Autodesk Fusion 360 part; units mm, degrees
(part 2 of 23)
  line L148 (51.3842, 29.2749) -> (51.3842, 29.6644)
  arc A510 (53.5996, 31.1037) -> (53.5996, 31.0529) centre (53.5996, 31.0783) ccw
  line L149 (53.9242, 28.6399) -> (53.9242, 28.2504)
  arc A511 (52.7812, 28.6399) -> (52.7304, 28.6399) centre (52.7558, 28.6399) ccw
  arc A512 (53.9365, 29.8369) -> (53.9119, 29.8813) centre (53.9242, 29.8591) ccw
  arc A513 (53.9496, 28.6399) -> (53.8988, 28.6399) centre (53.9242, 28.6399) ccw
  arc A514 (52.7812, 28.2504) -> (52.7304, 28.2504) centre (52.7558, 28.2504) ccw
  arc A515 (53.9496, 28.2504) -> (53.8988, 28.2504) centre (53.9242, 28.2504) ccw
  arc A516 (37.4142, 29.5233) -> (36.7651, 29.5233) centre (37.0896, 29.5233) ccw
  arc A517 (36.2204, 29.5882) -> (36.2712, 29.5882) centre (36.2458, 29.5882) ccw
  arc A518 (53.8988, 28.2504) -> (53.9496, 28.2504) centre (53.9242, 28.2504) ccw
  arc A519 (36.7651, 29.5882) -> (36.2458, 29.5882) centre (36.5055, 29.5882) ccw
  arc A520 (36.7905, 29.5882) -> (36.7397, 29.5882) centre (36.7651, 29.5882) ccw
  arc A521 (53.9242, 28.6145) -> (53.9242, 28.6653) centre (53.9242, 28.6399) ccw
  line L150 (53.2751, 28.4452) -> (53.2751, 28.6399)
  arc A522 (53.2497, 28.4452) -> (53.3005, 28.4452) centre (53.2751, 28.4452) ccw
  arc A523 (53.6646, 27.9654) -> (53.6646, 28.0162) centre (53.6646, 27.9908) ccw
  arc A524 (37.0967, 28.0882) -> (37.1475, 28.0882) centre (37.1221, 28.0882) ccw
  line L151 (53.9242, 29.21) -> (52.7558, 29.21)
  line L152 (53.9242, 30.4292) -> (52.7558, 30.4292)
  line L153 (52.7558, 29.21) -> (53.9242, 29.8591)
  line L154 (53.9242, 29.8591) -> (52.7558, 29.8591)
  line L155 (53.2751, 28.6399) -> (53.9242, 28.6399)
  arc A525 (52.7558, 29.8845) -> (52.7558, 29.8337) centre (52.7558, 29.8591) ccw
  arc A526 (53.9242, 29.8337) -> (53.9242, 29.8845) centre (53.9242, 29.8591) ccw
  arc A527 (36.2712, 29.5882) -> (36.2204, 29.5882) centre (36.2458, 29.5882) ccw
  arc A528 (53.6646, 28.0162) -> (53.6646, 27.9654) centre (53.6646, 27.9908) ccw
  arc A529 (53.9242, 29.1846) -> (53.9242, 29.2354) centre (53.9242, 29.21) ccw
  line L156 (37.4142, 29.1987) -> (37.4142, 29.5233)
  arc A530 (36.7397, 29.5882) -> (36.7905, 29.5882) centre (36.7651, 29.5882) ccw
  arc A531 (36.7397, 29.5233) -> (36.7905, 29.5233) centre (36.7651, 29.5233) ccw
  line L157 (36.7651, 29.5882) -> (36.7651, 29.3285)
  line L158 (52.7558, 30.4292) -> (52.7558, 30.7537)
  arc A532 (52.7812, 30.7537) -> (52.7304, 30.7537) centre (52.7558, 30.7537) ccw
  arc A533 (36.2204, 29.1987) -> (36.2712, 29.1987) centre (36.2458, 29.1987) ccw
  line L159 (52.7558, 28.2504) -> (52.7558, 28.6399)
  arc A534 (52.7304, 30.4292) -> (52.7812, 30.4292) centre (52.7558, 30.4292) ccw
  line L160 (53.0804, 31.0783) -> (53.5996, 31.0783)
  arc A535 (53.6646, 27.9908) -> (53.9242, 28.2504) centre (53.6646, 28.2504) ccw
  arc A536 (53.2751, 28.6653) -> (53.2751, 28.6145) centre (53.2751, 28.6399) ccw
  arc A537 (52.7558, 30.4546) -> (52.7558, 30.4038) centre (52.7558, 30.4292) ccw
  line L161 (53.6646, 27.9908) -> (53.0154, 27.9908)
  arc A538 (51.3588, 29.2749) -> (51.4096, 29.2749) centre (51.3842, 29.2749) ccw
  line L162 (55.3085, 2.4892) -> (55.9576, 2.4892)
  arc A539 (59.4599, 1.2954) -> (59.4599, 1.3462) centre (59.4599, 1.3208) ccw
  arc A540 (58.1499, 1.5804) -> (58.0991, 1.5804) centre (58.1245, 1.5804) ccw
  line L163 (50.9298, 27.9908) -> (50.9298, 28.7697)
  arc A541 (57.3644, 1.8655) -> (57.3644, 1.8147) centre (57.3644, 1.8401) ccw
  arc A542 (59.4599, 1.3462) -> (59.4599, 1.2954) centre (59.4599, 1.3208) ccw
  arc A543 (58.0991, 1.5804) -> (58.1499, 1.5804) centre (58.1245, 1.5804) ccw
  arc A544 (61.5711, 2.4812) -> (61.5229, 2.4972) centre (61.547, 2.4892) ccw
  arc A545 (55.3085, 2.5146) -> (55.3085, 2.4638) centre (55.3085, 2.4892) ccw
  arc A546 (59.4599, 2.4638) -> (59.4599, 2.5146) centre (59.4599, 2.4892) ccw
  arc A547 (57.3644, 2.4638) -> (57.3644, 2.5146) centre (57.3644, 2.4892) ccw
  arc A548 (55.9576, 2.4638) -> (55.9576, 2.5146) centre (55.9576, 2.4892) ccw
  line L164 (61.1575, 1.3208) -> (61.547, 2.4892)
  arc A549 (59.1354, 2.5146) -> (59.1354, 2.4638) centre (59.1354, 2.4892) ccw
  line L165 (58.6438, 1.3208) -> (58.3842, 1.3208)
  line L166 (57.0399, 1.3208) -> (57.0399, 2.4892)
  arc A550 (58.3842, 1.3462) -> (58.3842, 1.2954) centre (58.3842, 1.3208) ccw
  line L167 (58.3842, 2.4892) -> (58.6438, 2.4892)
  arc A551 (59.1608, 2.4892) -> (59.11, 2.4892) centre (59.1354, 2.4892) ccw
  arc A552 (61.976, 1.3462) -> (61.976, 1.2954) centre (61.976, 1.3208) ccw
  arc A553 (59.4599, 1.9953) -> (59.4599, 1.9445) centre (59.4599, 1.9699) ccw
  line L168 (51.3193, 28.3803) -> (50.5404, 28.3803)
  arc A554 (50.5404, 28.4057) -> (50.5404, 28.3549) centre (50.5404, 28.3803) ccw
  arc A555 (59.4599, 1.9953) -> (59.4599, 1.9445) centre (59.4599, 1.9699) ccw
  arc A556 (61.1334, 1.3288) -> (61.1816, 1.3128) centre (61.1575, 1.3208) ccw
  arc A557 (57.3644, 1.8401) -> (57.3644, 2.4892) centre (57.3644, 2.1646) ccw
  arc A558 (58.6438, 2.4638) -> (58.6438, 2.5146) centre (58.6438, 2.4892) ccw
  arc A559 (62.3005, 1.3208) -> (62.3005, 1.9699) centre (62.3005, 1.6453) ccw
  line L169 (57.0399, 2.4892) -> (57.3644, 2.4892)
  line L170 (59.1354, 2.4892) -> (59.4599, 2.4892)
  arc A560 (62.3005, 1.2954) -> (62.3005, 1.3462) centre (62.3005, 1.3208) ccw
  line L171 (59.1354, 1.3208) -> (59.1354, 2.4892)
  line L172 (59.4599, 1.3208) -> (59.1354, 1.3208)
  arc A561 (59.1354, 1.3462) -> (59.1354, 1.2954) centre (59.1354, 1.3208) ccw
  arc A562 (59.11, 1.3208) -> (59.1608, 1.3208) centre (59.1354, 1.3208) ccw
  line L173 (58.1245, 1.5804) -> (58.1245, 2.2296)
  arc A563 (51.4096, 29.6644) -> (51.3588, 29.6644) centre (51.3842, 29.6644) ccw
  arc A564 (51.3842, 29.6644) -> (51.1246, 29.924) centre (51.1246, 29.6644) ccw
  arc A565 (59.4599, 2.5146) -> (59.4599, 2.4638) centre (59.4599, 2.4892) ccw
  arc A566 (50.9044, 27.9908) -> (50.9552, 27.9908) centre (50.9298, 27.9908) ccw
  arc A567 (58.0991, 2.2296) -> (58.1499, 2.2296) centre (58.1245, 2.2296) ccw
  arc A568 (58.1499, 2.2296) -> (58.0991, 2.2296) centre (58.1245, 2.2296) ccw
  arc A569 (57.0653, 2.4892) -> (57.0145, 2.4892) centre (57.0399, 2.4892) ccw
  arc A570 (60.7921, 2.4972) -> (60.7439, 2.4812) centre (60.768, 2.4892) ccw
  arc A571 (57.0145, 1.3208) -> (57.0653, 1.3208) centre (57.0399, 1.3208) ccw
  arc A572 (50.9552, 28.7697) -> (50.9044, 28.7697) centre (50.9298, 28.7697) ccw
  arc A573 (59.4599, 1.3208) -> (59.4599, 1.9699) centre (59.4599, 1.6453) ccw
  arc A574 (58.3842, 1.2954) -> (58.3842, 1.3462) centre (58.3842, 1.3208) ccw
  arc A575 (59.1354, 1.9953) -> (59.1354, 1.9445) centre (59.1354, 1.9699) ccw
  arc A576 (58.3842, 2.4892) -> (58.1245, 2.2296) centre (58.3842, 2.2295) ccw
  arc A577 (57.3644, 1.8147) -> (57.3644, 1.8655) centre (57.3644, 1.8401) ccw
  arc A578 (55.6076, 1.3208) -> (55.6584, 1.3208) centre (55.633, 1.3208) ccw
  arc A579 (51.3193, 28.3549) -> (51.3193, 28.4057) centre (51.3193, 28.3803) ccw
  arc A580 (58.3842, 2.4638) -> (58.3842, 2.5146) centre (58.3842, 2.4892) ccw
  arc A581 (59.4599, 1.9699) -> (59.4599, 2.4892) centre (59.4599, 2.2296) ccw
  arc A582 (51.3588, 29.6644) -> (51.4096, 29.6644) centre (51.3842, 29.6644) ccw
  arc A583 (59.4599, 1.9445) -> (59.4599, 1.9953) centre (59.4599, 1.9699) ccw
  line L174 (54.4288, 1.5804) -> (54.4288, 2.2296)
  arc A584 (53.4819, 2.5146) -> (53.4819, 2.4638) centre (53.4819, 2.4892) ccw
  line L175 (57.3644, 1.8401) -> (57.0399, 1.8401)
  line L176 (59.1354, 1.9699) -> (59.4599, 1.9699)
  line L177 (60.768, 2.4892) -> (61.1575, 1.3208)
  arc A585 (57.3644, 2.5146) -> (57.3644, 2.4638) centre (57.3644, 2.4892) ccw
  line L178 (6.3585, 1.1938) -> (6.7479, 2.3622)
  arc A586 (57.0399, 1.8655) -> (57.0399, 1.8147) centre (57.0399, 1.8401) ccw
  line L179 (5.969, 2.3622) -> (6.3585, 1.1938)
  arc A587 (13.9023, 1.1938) -> (13.9531, 1.1938) centre (13.9277, 1.1938) ccw
  arc A588 (12.9892, 1.1858) -> (13.0374, 1.2018) centre (13.0133, 1.1938) ccw
  arc A589 (14.0575, 1.1684) -> (14.0575, 1.2192) centre (14.0575, 1.1938) ccw
  line L180 (5.54, 1.4534) -> (5.54, 1.5833)
  line L181 (13.7978, 1.1938) -> (14.0575, 1.1938)
  arc A590 (62.3654, 1.9445) -> (62.3654, 1.9953) centre (62.3654, 1.9699) ccw
  arc A591 (4.8655, 1.8429) -> (4.9163, 1.8429) centre (4.8909, 1.8429) ccw
  arc A592 (13.4268, 2.3542) -> (13.3786, 2.3702) centre (13.4027, 2.3622) ccw
  line L182 (13.7978, 2.3622) -> (14.0575, 2.3622)
  arc A593 (57.0399, 2.5146) -> (57.0399, 2.4638) centre (57.0399, 2.4892) ccw
  arc A594 (14.0575, 2.3368) -> (14.0575, 2.3876) centre (14.0575, 2.3622) ccw
  line L183 (4.8909, 1.8429) -> (4.8909, 2.3622)
  arc A595 (5.2804, 1.8683) -> (5.2804, 1.8175) centre (5.2804, 1.8429) ccw
  arc A596 (5.5654, 1.4534) -> (5.5146, 1.4534) centre (5.54, 1.4534) ccw
  arc A597 (5.54, 2.3368) -> (5.54, 2.3876) centre (5.54, 2.3622) ccw
  line L184 (14.5556, 1.1938) -> (14.5556, 2.3622)
  arc A598 (4.8909, 1.2192) -> (4.8909, 1.1684) centre (4.8909, 1.1938) ccw
  arc A599 (14.581, 2.3622) -> (14.5302, 2.3622) centre (14.5556, 2.3622) ccw
  line L185 (61.976, 1.3208) -> (62.3005, 1.3208)
  arc A600 (5.5146, 1.5833) -> (5.5654, 1.5833) centre (5.54, 1.5833) ccw
  line L186 (4.8909, 2.3622) -> (5.54, 2.3622)
  arc A601 (5.2804, 1.8175) -> (5.2804, 1.8683) centre (5.2804, 1.8429) ccw
  arc A602 (62.1058, 1.9953) -> (62.1058, 1.9445) centre (62.1058, 1.9699) ccw
  line L187 (13.9277, 2.3622) -> (13.9277, 1.1938)
  arc A603 (62.3654, 1.9953) -> (62.3654, 1.9445) centre (62.3654, 1.9699) ccw
  arc A604 (61.976, 2.5146) -> (61.976, 2.4638) centre (61.976, 2.4892) ccw
  arc A605 (5.2804, 1.2192) -> (5.2804, 1.1684) centre (5.2804, 1.1938) ccw
  arc A606 (5.2804, 1.1938) -> (5.54, 1.4534) centre (5.2804, 1.4534) ccw
  line L188 (3.9963, 1.2587) -> (3.9963, 2.0376)
  arc A607 (3.6068, 1.6736) -> (3.6068, 1.6228) centre (3.6068, 1.6482) ccw
  arc A608 (58.6438, 1.2954) -> (58.6438, 1.3462) centre (58.6438, 1.3208) ccw
  arc A609 (4.8909, 1.8683) -> (4.8909, 1.8175) centre (4.8909, 1.8429) ccw
  arc A610 (6.3344, 1.1858) -> (6.3826, 1.2018) centre (6.3585, 1.1938) ccw
  arc A611 (13.7978, 1.2192) -> (13.7978, 1.1684) centre (13.7978, 1.1938) ccw
  arc A612 (5.54, 1.5833) -> (5.2804, 1.8429) centre (5.2804, 1.5833) ccw
  arc A613 (12.6479, 2.3702) -> (12.5997, 2.3542) centre (12.6238, 2.3622) ccw
  arc A614 (14.5778, 2.3745) -> (14.5334, 2.3499) centre (14.5556, 2.3622) ccw
  arc A615 (5.5146, 1.4534) -> (5.5654, 1.4534) centre (5.54, 1.4534) ccw
  line L189 (61.976, 2.4892) -> (62.3654, 2.4892)
  arc A616 (6.772, 2.3542) -> (6.7238, 2.3702) centre (6.7479, 2.3622) ccw
  arc A617 (5.2804, 1.1684) -> (5.2804, 1.2192) centre (5.2804, 1.1938) ccw
  line L190 (13.0133, 1.1938) -> (13.4027, 2.3622)
  arc A618 (61.1334, 1.3128) -> (61.1816, 1.3288) centre (61.1575, 1.3208) ccw
  arc A619 (4.0217, 2.0376) -> (3.9709, 2.0376) centre (3.9963, 2.0376) ccw
  arc A620 (4.9163, 2.3622) -> (4.8655, 2.3622) centre (4.8909, 2.3622) ccw
  arc A621 (4.3857, 1.6228) -> (4.3857, 1.6736) centre (4.3857, 1.6482) ccw
  arc A622 (5.5654, 1.5833) -> (5.5146, 1.5833) centre (5.54, 1.5833) ccw
  arc A623 (58.1245, 1.5804) -> (58.3842, 1.3208) centre (58.3842, 1.5805) ccw
  arc A624 (62.3005, 1.9953) -> (62.3005, 1.9445) centre (62.3005, 1.9699) ccw
  arc A625 (4.8909, 2.3876) -> (4.8909, 2.3368) centre (4.8909, 2.3622) ccw
  arc A626 (62.3654, 2.4638) -> (62.3654, 2.5146) centre (62.3654, 2.4892) ccw
  arc A627 (58.3842, 2.5146) -> (58.3842, 2.4638) centre (58.3842, 2.4892) ccw
  arc A628 (3.9709, 1.2587) -> (4.0217, 1.2587) centre (3.9963, 1.2587) ccw
  arc A629 (5.9931, 2.3702) -> (5.9449, 2.3542) centre (5.969, 2.3622) ccw
  line L191 (3.6068, 1.6482) -> (4.3857, 1.6482)
  arc A630 (6.3344, 1.2018) -> (6.3826, 1.1858) centre (6.3585, 1.1938) ccw
  arc A631 (62.3005, 1.3462) -> (62.3005, 1.2954) centre (62.3005, 1.3208) ccw
  arc A632 (62.3654, 1.9699) -> (62.3654, 2.4892) centre (62.3654, 2.2296) ccw
  line L192 (4.8909, 1.1938) -> (5.2804, 1.1938)
  arc A633 (12.9892, 1.2018) -> (13.0374, 1.1858) centre (13.0133, 1.1938) ccw
  line L193 (5.2804, 1.8429) -> (4.8909, 1.8429)
  arc A634 (40.3154, 19.1262) -> (40.3154, 19.0754) centre (40.3154, 19.1008) ccw
  arc A635 (41.2496, 19.7499) -> (41.1988, 19.7499) centre (41.2242, 19.7499) ccw
  arc A636 (22.7951, 20.3595) -> (22.7951, 20.4103) centre (22.7951, 20.3849) ccw
  arc A637 (15.1793, 1.1938) -> (15.2301, 1.1938) centre (15.2047, 1.1938) ccw
  arc A638 (13.7978, 2.3876) -> (13.7978, 2.3368) centre (13.7978, 2.3622) ccw
  line L194 (40.0558, 20.32) -> (41.2242, 20.9691)
  arc A639 (40.5497, 19.5552) -> (40.6005, 19.5552) centre (40.5751, 19.5552) ccw
  arc A640 (23.4696, 20.7744) -> (23.4188, 20.7744) centre (23.4442, 20.7744) ccw
  arc A641 (40.3154, 19.0754) -> (40.3154, 19.1262) centre (40.3154, 19.1008) ccw
  arc A642 (40.9646, 19.1008) -> (41.2242, 19.3604) centre (40.9646, 19.3604) ccw
  arc A643 (23.4362, 21.8284) -> (23.4522, 21.8766) centre (23.4442, 21.8525) ccw
  line L195 (41.2242, 20.9691) -> (40.0558, 20.9691)
  arc A644 (22.6004, 19.5157) -> (22.6004, 19.4649) centre (22.6004, 19.4903) ccw
  line L196 (22.7951, 20.3849) -> (22.2758, 20.3849)
  line L197 (22.9898, 19.1008) -> (22.9898, 19.8797)
  line L198 (14.5556, 2.3622) -> (15.2047, 1.1938)
  arc A645 (40.0558, 20.9945) -> (40.0558, 20.9437) centre (40.0558, 20.9691) ccw
  arc A646 (41.2242, 19.7245) -> (41.2242, 19.7753) centre (41.2242, 19.7499) ccw
  arc A647 (23.4188, 20.7744) -> (23.4696, 20.7744) centre (23.4442, 20.7744) ccw
  arc A648 (40.0558, 19.3604) -> (40.3154, 19.1008) centre (40.3154, 19.3604) ccw
  line L199 (23.1846, 21.034) -> (23.0547, 21.034)
  arc A649 (40.0812, 19.7499) -> (40.0304, 19.7499) centre (40.0558, 19.7499) ccw
  arc A650 (40.0304, 19.3604) -> (40.0812, 19.3604) centre (40.0558, 19.3604) ccw
  arc A651 (23.4188, 20.3849) -> (23.4696, 20.3849) centre (23.4442, 20.3849) ccw
  arc A652 (41.2496, 19.3604) -> (41.1988, 19.3604) centre (41.2242, 19.3604) ccw
  arc A653 (40.9646, 19.1262) -> (40.9646, 19.0754) centre (40.9646, 19.1008) ccw
  arc A654 (40.0812, 19.3604) -> (40.0304, 19.3604) centre (40.0558, 19.3604) ccw
  arc A655 (23.1846, 21.0086) -> (23.1846, 21.0594) centre (23.1846, 21.034) ccw
  arc A656 (22.2838, 22.266) -> (22.2678, 22.2178) centre (22.2758, 22.2419) ccw
  arc A657 (22.3012, 21.034) -> (22.2504, 21.034) centre (22.2758, 21.034) ccw
  arc A658 (40.9646, 19.0754) -> (40.9646, 19.1262) centre (40.9646, 19.1008) ccw
  line L200 (41.2242, 20.32) -> (40.0558, 20.32)
  arc A659 (22.8205, 20.7744) -> (22.7697, 20.7744) centre (22.7951, 20.7744) ccw
  arc A660 (22.2504, 20.3849) -> (22.3012, 20.3849) centre (22.2758, 20.3849) ccw
  arc A661 (22.2758, 20.4103) -> (22.2758, 20.3595) centre (22.2758, 20.3849) ccw
  arc A662 (23.1846, 21.0594) -> (23.1846, 21.0086) centre (23.1846, 21.034) ccw
  arc A663 (22.7697, 20.3849) -> (22.8205, 20.3849) centre (22.7951, 20.3849) ccw
  arc A664 (14.5302, 1.1938) -> (14.581, 1.1938) centre (14.5556, 1.1938) ccw
  arc A665 (62.3654, 2.5146) -> (62.3654, 2.4638) centre (62.3654, 2.4892) ccw
  line L201 (40.5751, 19.5552) -> (40.5751, 19.7499)
  arc A666 (15.2301, 2.3622) -> (15.1793, 2.3622) centre (15.2047, 2.3622) ccw
  arc A667 (22.9644, 19.1008) -> (23.0152, 19.1008) centre (22.9898, 19.1008) ccw
  arc A668 (23.4522, 21.8284) -> (23.4362, 21.8766) centre (23.4442, 21.8525) ccw
  arc A669 (40.5751, 19.7753) -> (40.5751, 19.7245) centre (40.5751, 19.7499) ccw
  line L202 (40.0558, 19.3604) -> (40.0558, 19.7499)
  line L203 (40.9646, 19.1008) -> (40.3154, 19.1008)
  line L204 (23.4442, 21.8525) -> (22.2758, 22.2419)
  arc A670 (22.7697, 20.7744) -> (22.8205, 20.7744) centre (22.7951, 20.7744) ccw
  arc A671 (40.6005, 19.7499) -> (40.5497, 19.7499) centre (40.5751, 19.7499) ccw
  line L205 (62.3654, 1.9699) -> (62.1058, 1.9699)
  arc A672 (23.0547, 21.0594) -> (23.0547, 21.0086) centre (23.0547, 21.034) ccw
  arc A673 (41.1988, 19.3604) -> (41.2496, 19.3604) centre (41.2242, 19.3604) ccw
  arc A674 (40.0435, 20.3422) -> (40.0681, 20.2978) centre (40.0558, 20.32) ccw
  line L206 (22.2758, 20.3849) -> (22.2758, 21.034)
  arc A675 (13.9531, 2.3622) -> (13.9023, 2.3622) centre (13.9277, 2.3622) ccw
  line L207 (23.3793, 19.4903) -> (22.6004, 19.4903)
  line L208 (23.4442, 20.3849) -> (23.4442, 20.7744)
  line L209 (12.6238, 2.3622) -> (13.0133, 1.1938)
  line L210 (15.2047, 1.1938) -> (15.2047, 2.3622)
  line L211 (41.2242, 19.7499) -> (41.2242, 19.3604)
  arc A676 (22.2678, 21.4871) -> (22.2838, 21.4389) centre (22.2758, 21.463) ccw
  arc A677 (15.1825, 1.1815) -> (15.2269, 1.2061) centre (15.2047, 1.1938) ccw
  arc A678 (23.4442, 20.7744) -> (23.1846, 21.034) centre (23.1846, 20.7744) ccw
  line L212 (22.2758, 21.463) -> (23.4442, 21.8525)
  arc A679 (41.1988, 52.5018) -> (41.2496, 52.5018) centre (41.2242, 52.5018) ccw
  line L213 (27.1893, 28.3803) -> (26.4104, 28.3803)
  line L214 (28.9504, 31.0783) -> (29.4696, 31.0783)
  arc A680 (24.8035, 54.4558) -> (24.8281, 54.4114) centre (24.8158, 54.4336) ccw
  arc A681 (24.8158, 55.1081) -> (24.8158, 55.0573) centre (24.8158, 55.0827) ccw
  arc A682 (27.2796, 29.6644) -> (27.2288, 29.6644) centre (27.2542, 29.6644) ccw
  line L215 (27.2542, 29.2749) -> (27.2542, 29.6644)
  arc A683 (27.2288, 29.2749) -> (27.2796, 29.2749) centre (27.2542, 29.2749) ccw
  arc A684 (27.2542, 29.6644) -> (26.9946, 29.924) centre (26.9946, 29.6644) ccw
  arc A685 (25.9842, 55.0573) -> (25.9842, 55.1081) centre (25.9842, 55.0827) ccw
  arc A686 (26.8252, 28.7697) -> (26.7744, 28.7697) centre (26.7998, 28.7697) ccw
  arc A687 (26.4104, 28.4057) -> (26.4104, 28.3549) centre (26.4104, 28.3803) ccw
  line L216 (26.9946, 29.924) -> (26.8647, 29.924)
  arc A688 (26.9946, 29.9494) -> (26.9946, 29.8986) centre (26.9946, 29.924) ccw
  line L217 (25.9842, 55.0827) -> (24.8158, 55.0827)
  line L218 (29.5346, 27.9908) -> (28.8854, 27.9908)
  arc A689 (26.0858, 29.3003) -> (26.0858, 29.2495) centre (26.0858, 29.2749) ccw
  arc A690 (40.2956, 53.667) -> (40.3353, 53.6988) centre (40.3154, 53.6829) ccw
  arc A691 (26.0938, 31.156) -> (26.0778, 31.1078) centre (26.0858, 31.1319) ccw
  arc A692 (29.5346, 28.0162) -> (29.5346, 27.9654) centre (29.5346, 27.9908) ccw
  line L219 (26.7998, 27.9908) -> (26.7998, 28.7697)
  arc A693 (27.1893, 28.3549) -> (27.1893, 28.4057) centre (27.1893, 28.3803) ccw
  arc A694 (26.7744, 27.9908) -> (26.8252, 27.9908) centre (26.7998, 27.9908) ccw
  arc A695 (27.2462, 30.7184) -> (27.2622, 30.7666) centre (27.2542, 30.7425) ccw
  arc A696 (27.2288, 29.6644) -> (27.2796, 29.6644) centre (27.2542, 29.6644) ccw
  arc A697 (25.9965, 55.0605) -> (25.9719, 55.1049) centre (25.9842, 55.0827) ccw
  arc A698 (40.0756, 54.0233) -> (40.036, 53.9916) centre (40.0558, 54.0075) ccw
  line L220 (33.6042, 53.6829) -> (33.6042, 54.332)
  arc A699 (41.2496, 52.8264) -> (41.1988, 52.8264) centre (41.2242, 52.8264) ccw
  arc A700 (29.1197, 28.4452) -> (29.1705, 28.4452) centre (29.1451, 28.4452) ccw
  line L221 (32.4358, 52.5018) -> (32.4358, 52.8264)
  line L222 (33.6042, 52.8264) -> (33.6042, 52.5018)
  arc A701 (33.6042, 55.1504) -> (32.9551, 55.1504) centre (33.2797, 55.1504) ccw
  arc A702 (32.9297, 55.1504) -> (32.9805, 55.1504) centre (32.9551, 55.1504) ccw
  arc A703 (40.2098, 54.8992) -> (40.2263, 54.9473) centre (40.2181, 54.9233) ccw
  line L223 (32.4358, 54.8259) -> (32.4358, 55.2154)
  line L224 (36.1442, 52.5018) -> (34.9758, 52.5018)
  arc A704 (32.4104, 55.2154) -> (32.4612, 55.2154) centre (32.4358, 55.2154) ccw
  arc A705 (36.1442, 52.4764) -> (36.1442, 52.5272) centre (36.1442, 52.5018) ccw
  arc A706 (40.0558, 54.0329) -> (40.0558, 53.9821) centre (40.0558, 54.0075) ccw
  arc A707 (33.2796, 53.1255) -> (33.2796, 53.1763) centre (33.2796, 53.1509) ccw
  arc A708 (32.7604, 53.1763) -> (32.7604, 53.1255) centre (32.7604, 53.1509) ccw
  arc A709 (33.2796, 53.1763) -> (33.2796, 53.1255) centre (33.2796, 53.1509) ccw
  arc A710 (33.5788, 52.8264) -> (33.6296, 52.8264) centre (33.6042, 52.8264) ccw
  arc A711 (32.4556, 54.0233) -> (32.416, 53.9916) centre (32.4358, 54.0075) ccw
  arc A712 (33.6296, 55.1504) -> (33.5788, 55.1504) centre (33.6042, 55.1504) ccw
  arc A713 (26.8647, 29.924) -> (26.6051, 29.6644) centre (26.8647, 29.6644) ccw
  arc A714 (32.4104, 52.5018) -> (32.4612, 52.5018) centre (32.4358, 52.5018) ccw
  arc A715 (40.0812, 55.1504) -> (40.0304, 55.1504) centre (40.0558, 55.1504) ccw
  arc A716 (32.4612, 52.8264) -> (32.4104, 52.8264) centre (32.4358, 52.8264) ccw
  line L225 (32.7604, 53.1509) -> (33.2796, 53.1509)
  line L226 (32.4358, 54.0075) -> (33.6042, 54.0075)
  line L227 (41.2242, 53.6829) -> (41.2242, 54.332)
  arc A717 (33.6296, 54.332) -> (33.5788, 54.332) centre (33.6042, 54.332) ccw
  arc A718 (32.4104, 54.8259) -> (32.4612, 54.8259) centre (32.4358, 54.8259) ccw
  arc A719 (40.2181, 55.3776) -> (40.0558, 55.1504) centre (40.296, 55.1504) ccw
  arc A720 (33.5788, 52.5018) -> (33.6296, 52.5018) centre (33.6042, 52.5018) ccw
  arc A721 (32.9551, 55.2154) -> (32.4358, 55.2154) centre (32.6955, 55.2154) ccw
  line L228 (33.6042, 54.8259) -> (33.6042, 55.1504)
  line L229 (40.3154, 53.6829) -> (40.0558, 54.0075)
  line L230 (40.0558, 54.0075) -> (41.2242, 54.0075)
  arc A722 (33.6042, 52.4764) -> (33.6042, 52.5272) centre (33.6042, 52.5018) ccw
  arc A723 (33.5788, 54.8259) -> (33.6296, 54.8259) centre (33.6042, 54.8259) ccw
  arc A724 (32.4358, 52.5272) -> (32.4358, 52.4764) centre (32.4358, 52.5018) ccw
  arc A725 (32.9297, 55.2154) -> (32.9805, 55.2154) centre (32.9551, 55.2154) ccw
  arc A726 (41.2242, 53.9821) -> (41.2242, 54.0329) centre (41.2242, 54.0075) ccw
  arc A727 (33.5788, 55.1504) -> (33.6296, 55.1504) centre (33.6042, 55.1504) ccw
  arc A728 (54.4034, 1.5804) -> (54.4542, 1.5804) centre (54.4288, 1.5804) ccw
  arc A729 (32.9297, 54.9557) -> (32.9805, 54.9557) centre (32.9551, 54.9557) ccw
  arc A730 (32.4104, 52.8264) -> (32.4612, 52.8264) centre (32.4358, 52.8264) ccw
  arc A731 (34.9758, 52.5272) -> (34.9758, 52.4764) centre (34.9758, 52.5018) ccw
  arc A732 (32.4612, 55.2154) -> (32.4104, 55.2154) centre (32.4358, 55.2154) ccw
  arc A733 (40.64, 54.8005) -> (40.64, 54.8513) centre (40.64, 54.8259) ccw
  arc A734 (29.7942, 28.6145) -> (29.7942, 28.6653) centre (29.7942, 28.6399) ccw
  arc A735 (32.7604, 53.1255) -> (32.7604, 53.1763) centre (32.7604, 53.1509) ccw
  arc A736 (32.6756, 53.667) -> (32.7153, 53.6988) centre (32.6955, 53.6829) ccw
  arc A737 (32.4358, 54.0329) -> (32.4358, 53.9821) centre (32.4358, 54.0075) ccw
  arc A738 (41.2496, 54.332) -> (41.1988, 54.332) centre (41.2242, 54.332) ccw
  arc A739 (40.0558, 55.1504) -> (40.2181, 54.9233) centre (40.2959, 55.1504) ccw
  arc A740 (33.6296, 52.8264) -> (33.5788, 52.8264) centre (33.6042, 52.8264) ccw
  line L231 (32.6954, 53.6829) -> (32.4358, 54.0075)
  arc A741 (40.2181, 54.9233) -> (40.64, 54.8259) centre (40.6401, 55.7886) ccw
  arc A742 (41.1988, 53.6829) -> (41.2496, 53.6829) centre (41.2242, 53.6829) ccw
  arc A743 (26.1112, 29.924) -> (26.0604, 29.924) centre (26.0858, 29.924) ccw
  arc A744 (32.7604, 53.1509) -> (32.4358, 52.8264) centre (32.7604, 52.8263) ccw
  arc A745 (33.6042, 52.8264) -> (33.2796, 53.1509) centre (33.2796, 52.8263) ccw
  arc A746 (40.2292, 54.9461) -> (40.2069, 54.9004) centre (40.2181, 54.9233) ccw
  arc A747 (33.6042, 53.9821) -> (33.6042, 54.0329) centre (33.6042, 54.0075) ccw
  arc A748 (32.9805, 55.2154) -> (32.9297, 55.2154) centre (32.9551, 55.2154) ccw
  arc A749 (33.5788, 53.6829) -> (33.6296, 53.6829) centre (33.6042, 53.6829) ccw
  line L232 (32.9551, 55.2154) -> (32.9551, 54.9557)
  line L233 (36.1442, 52.8264) -> (36.1442, 52.5018)
  line L234 (34.9758, 52.5018) -> (34.9758, 52.8264)
  arc A750 (36.1696, 52.8264) -> (36.1188, 52.8264) centre (36.1442, 52.8264) ccw
  arc A751 (36.1277, 54.8065) -> (36.1607, 54.8452) centre (36.1442, 54.8258) ccw
  arc A752 (37.8404, 53.1509) -> (37.5158, 52.8264) centre (37.8404, 52.8263) ccw
  arc A753 (36.1442, 52.8264) -> (35.8196, 53.1509) centre (35.8196, 52.8263) ccw
  arc A754 (34.9956, 54.0233) -> (34.956, 53.9916) centre (34.9758, 54.0074) ccw
  arc A755 (38.3596, 53.1763) -> (38.3596, 53.1255) centre (38.3596, 53.1509) ccw
  arc A756 (35.3004, 53.1509) -> (34.9758, 52.8264) centre (35.3004, 52.8263) ccw
  arc A757 (38.3596, 53.1255) -> (38.3596, 53.1763) centre (38.3596, 53.1509) ccw
  arc A758 (38.6842, 53.9821) -> (38.6842, 54.0329) centre (38.6842, 54.0075) ccw
  arc A759 (34.9504, 52.8264) -> (35.0012, 52.8264) centre (34.9758, 52.8264) ccw
  line L235 (35.4951, 55.3776) -> (36.1442, 54.8259)
  line L236 (37.7754, 54.8259) -> (37.5158, 55.1504)
  line L237 (35.3004, 53.1509) -> (35.8196, 53.1509)
  line L238 (37.5158, 52.5018) -> (37.5158, 52.8264)
  arc A760 (35.2679, 55.5004) -> (35.2679, 55.4496) centre (35.2679, 55.475) ccw
  arc A761 (36.1442, 53.9821) -> (36.1442, 54.0329) centre (36.1442, 54.0075) ccw
  arc A762 (37.5412, 52.8264) -> (37.4904, 52.8264) centre (37.5158, 52.8264) ccw
  line L239 (36.1442, 53.6829) -> (36.1442, 54.332)
  arc A763 (35.3004, 53.1763) -> (35.3004, 53.1255) centre (35.3004, 53.1509) ccw
  arc A764 (36.1188, 52.5018) -> (36.1696, 52.5018) centre (36.1442, 52.5018) ccw
  arc A765 (37.4904, 52.8264) -> (37.5412, 52.8264) centre (37.5158, 52.8264) ccw
  line L240 (38.6842, 52.8264) -> (38.6842, 52.5018)
  arc A766 (35.5115, 55.397) -> (35.4786, 55.3583) centre (35.495, 55.3777) ccw
  arc A767 (37.4904, 52.5018) -> (37.5412, 52.5018) centre (37.5158, 52.5018) ccw
  arc A768 (38.6588, 52.5018) -> (38.7096, 52.5018) centre (38.6842, 52.5018) ccw
  line L241 (37.5158, 54.0075) -> (38.6842, 54.0075)
  arc A769 (37.8404, 53.1255) -> (37.8404, 53.1763) centre (37.8404, 53.1509) ccw
  arc A770 (35.4951, 55.3776) -> (35.2679, 55.475) centre (35.2679, 55.1613) ccw
  line L242 (35.2354, 53.6829) -> (34.9758, 54.0075)
  arc A771 (38.6842, 52.4764) -> (38.6842, 52.5272) centre (38.6842, 52.5018) ccw
  arc A772 (37.8404, 53.1763) -> (37.8404, 53.1255) centre (37.8404, 53.1509) ccw
  arc A773 (35.8196, 53.1255) -> (35.8196, 53.1763) centre (35.8196, 53.1509) ccw
  arc A774 (36.1696, 54.332) -> (36.1188, 54.332) centre (36.1442, 54.332) ccw
  arc A775 (34.9504, 55.1829) -> (35.0012, 55.1829) centre (34.9758, 55.1829) ccw
  arc A776 (34.9758, 55.1829) -> (35.2354, 54.8259) centre (35.351, 55.1829) ccw
  arc A777 (34.9504, 52.5018) -> (35.0012, 52.5018) centre (34.9758, 52.5018) ccw
  line L243 (36.1442, 54.8259) -> (36.1442, 55.475)
  arc A778 (35.8196, 53.1763) -> (35.8196, 53.1255) centre (35.8196, 53.1509) ccw
  arc A779 (36.1188, 54.8259) -> (36.1696, 54.8259) centre (36.1442, 54.8259) ccw
  arc A780 (34.9758, 54.0329) -> (34.9758, 53.9821) centre (34.9758, 54.0075) ccw
  line L244 (34.9758, 54.0075) -> (36.1442, 54.0075)
  arc A781 (35.2679, 55.4496) -> (35.2679, 55.5004) centre (35.2679, 55.475) ccw
  arc A782 (36.1696, 55.475) -> (36.1188, 55.475) centre (36.1442, 55.475) ccw
  line L245 (38.6842, 52.5018) -> (37.5158, 52.5018)
  arc A783 (35.0012, 55.1829) -> (34.9504, 55.1829) centre (34.9758, 55.1829) ccw
  arc A784 (36.1188, 52.8264) -> (36.1696, 52.8264) centre (36.1442, 52.8264) ccw
  arc A785 (35.0012, 52.8264) -> (34.9504, 52.8264) centre (34.9758, 52.8264) ccw
  arc A786 (35.3004, 53.1255) -> (35.3004, 53.1763) centre (35.3004, 53.1509) ccw
  arc A787 (35.2679, 55.475) -> (34.9758, 55.1829) centre (35.2679, 55.1829) ccw
  arc A788 (35.4767, 55.3601) -> (35.5135, 55.3952) centre (35.4951, 55.3777) ccw
  arc A789 (37.5158, 52.5272) -> (37.5158, 52.4764) centre (37.5158, 52.5018) ccw
  arc A790 (36.1188, 53.6829) -> (36.1696, 53.6829) centre (36.1442, 53.6829) ccw
  line L246 (37.8404, 53.1509) -> (38.3596, 53.1509)
  arc A791 (38.7096, 52.8264) -> (38.6588, 52.8264) centre (38.6842, 52.8264) ccw
  arc A792 (38.6588, 52.8264) -> (38.7096, 52.8264) centre (38.6842, 52.8264) ccw
  arc A793 (38.6842, 52.8264) -> (38.3596, 53.1509) centre (38.3596, 52.8263) ccw
  arc A794 (37.5356, 54.0233) -> (37.496, 53.9916) centre (37.5158, 54.0074) ccw
  line L247 (37.7754, 53.6829) -> (37.5158, 54.0075)
  arc A795 (37.7556, 53.667) -> (37.7953, 53.6988) centre (37.7754, 53.6829) ccw
  arc A796 (35.2156, 53.667) -> (35.2553, 53.6988) centre (35.2355, 53.6829) ccw
  arc A797 (38.6588, 53.6829) -> (38.7096, 53.6829) centre (38.6842, 53.6829) ccw
  arc A798 (35.2276, 54.8017) -> (35.2433, 54.8501) centre (35.2355, 54.8259) ccw
  line L248 (37.5158, 55.1504) -> (38.6842, 55.1504)
  arc A799 (37.5158, 55.1758) -> (37.5158, 55.125) centre (37.5158, 55.1504) ccw
  arc A800 (38.7096, 54.332) -> (38.6588, 54.332) centre (38.6842, 54.332) ccw
  arc A801 (37.5356, 55.1663) -> (37.496, 55.1346) centre (37.5158, 55.1504) ccw
  arc A802 (37.7556, 54.81) -> (37.7953, 54.8418) centre (37.7754, 54.8259) ccw
  arc A803 (38.6842, 55.125) -> (38.6842, 55.1758) centre (38.6842, 55.1504) ccw
  line L249 (38.6842, 53.6829) -> (38.6842, 54.332)
  arc A804 (37.5158, 54.0329) -> (37.5158, 53.9821) centre (37.5158, 54.0075) ccw
  line L250 (41.2242, 52.5018) -> (40.0558, 52.5018)
  arc A805 (33.6804, 29.5557) -> (33.7312, 29.5557) centre (33.7058, 29.5557) ccw
  arc A806 (40.3804, 53.1255) -> (40.3804, 53.1763) centre (40.3804, 53.1509) ccw
  arc A807 (33.9979, 29.8478) -> (33.7058, 29.5557) centre (33.9979, 29.5557) ccw
  arc A808 (34.5567, 28.0882) -> (34.6075, 28.0882) centre (34.5821, 28.0882) ccw
  line L251 (38.6842, 54.8259) -> (38.6842, 55.475)
  line L252 (37.4974, 2.4892) -> (37.4974, 1.3208)
  arc A809 (38.6588, 54.8259) -> (38.7096, 54.8259) centre (38.6842, 54.8259) ccw
  arc A810 (40.0812, 52.8264) -> (40.0304, 52.8264) centre (40.0558, 52.8264) ccw
  arc A811 (41.2242, 52.4764) -> (41.2242, 52.5272) centre (41.2242, 52.5018) ccw
  arc A812 (40.3804, 53.1763) -> (40.3804, 53.1255) centre (40.3804, 53.1509) ccw
  line L253 (40.3804, 53.1509) -> (40.8996, 53.1509)
  line L254 (41.2242, 52.8264) -> (41.2242, 52.5018)
  arc A813 (34.6075, 28.6724) -> (34.5567, 28.6724) centre (34.5821, 28.6724) ccw
  arc A814 (40.0304, 52.8264) -> (40.0812, 52.8264) centre (40.0558, 52.8264) ccw
  arc A815 (40.3804, 53.1509) -> (40.0558, 52.8264) centre (40.3804, 52.8263) ccw
  arc A816 (41.2242, 52.8264) -> (40.8996, 53.1509) centre (40.8996, 52.8263) ccw
  arc A817 (37.157, 2.2494) -> (37.1888, 2.2097) centre (37.1729, 2.2296) ccw
  arc A818 (41.1988, 52.8264) -> (41.2496, 52.8264) centre (41.2242, 52.8264) ccw
  arc A819 (37.472, 1.3208) -> (37.5228, 1.3208) centre (37.4974, 1.3208) ccw
  line L255 (37.1729, 2.2296) -> (37.4974, 2.4892)
  arc A820 (37.1729, 1.3462) -> (37.1729, 1.2954) centre (37.1729, 1.3208) ccw
  line L256 (38.9636, 2.4892) -> (38.9636, 1.6454)
  arc A821 (34.8577, 29.1794) -> (34.8907, 29.2181) centre (34.8742, 29.1988) ccw
  arc A822 (37.5133, 2.4694) -> (37.4816, 2.509) centre (37.4975, 2.4892) ccw
  arc A823 (37.5228, 2.4892) -> (37.472, 2.4892) centre (37.4974, 2.4892) ccw
  line L257 (37.1729, 1.3208) -> (37.822, 1.3208)
  line L258 (40.0558, 52.5018) -> (40.0558, 52.8264)
  arc A824 (40.0304, 52.5018) -> (40.0812, 52.5018) centre (40.0558, 52.5018) ccw
  arc A825 (40.8996, 53.1763) -> (40.8996, 53.1255) centre (40.8996, 53.1509) ccw
  arc A826 (40.0558, 52.5272) -> (40.0558, 52.4764) centre (40.0558, 52.5018) ccw
  arc A827 (38.7096, 55.475) -> (38.6588, 55.475) centre (38.6842, 55.475) ccw
  arc A828 (40.8996, 53.1255) -> (40.8996, 53.1763) centre (40.8996, 53.1509) ccw
  arc A829 (33.9979, 29.8732) -> (33.9979, 29.8224) centre (33.9979, 29.8478) ccw
  arc A830 (38.9382, 1.6454) -> (38.989, 1.6454) centre (38.9636, 1.6454) ccw
  arc A831 (39.6381, 2.4892) -> (39.5873, 2.4892) centre (39.6127, 2.4892) ccw
  line L259 (39.6127, 1.6454) -> (39.6127, 2.4892)
  line L260 (44.8779, 1.3208) -> (44.6182, 1.8401)
  arc A832 (41.33, 2.5146) -> (41.33, 2.4638) centre (41.33, 2.4892) ccw
  arc A833 (45.3263, 1.4831) -> (45.7157, 1.3208) centre (45.7158, 1.8692) ccw
  arc A834 (41.5897, 2.4638) -> (41.5897, 2.5146) centre (41.5897, 2.4892) ccw
  line L261 (41.4598, 2.4892) -> (41.4598, 1.3208)
  line L262 (41.33, 2.4892) -> (41.5897, 2.4892)
  arc A835 (41.33, 1.3462) -> (41.33, 1.2954) centre (41.33, 1.3208) ccw
  arc A836 (40.2082, 2.4892) -> (40.1574, 2.4892) centre (40.1828, 2.4892) ccw
  arc A837 (37.822, 1.2954) -> (37.822, 1.3462) centre (37.822, 1.3208) ccw
  arc A838 (40.1574, 1.3208) -> (40.2082, 1.3208) centre (40.1828, 1.3208) ccw
  arc A839 (40.8065, 1.3208) -> (40.8573, 1.3208) centre (40.8319, 1.3208) ccw
  line L263 (42.3742, 1.3208) -> (42.7637, 2.4892)
  line L264 (43.233, 2.4892) -> (43.7523, 2.4892)
  line L265 (43.7523, 1.3208) -> (43.233, 1.3208)
  arc A840 (42.3501, 1.3288) -> (42.3983, 1.3128) centre (42.3742, 1.3208) ccw
  arc A841 (43.6225, 1.9445) -> (43.6225, 1.9953) centre (43.6225, 1.9699) ccw
  arc A842 (44.2033, 1.3208) -> (44.2541, 1.3208) centre (44.2287, 1.3208) ccw
  arc A843 (44.2287, 2.5146) -> (44.2287, 2.4638) centre (44.2287, 2.4892) ccw
  arc A844 (41.4852, 2.4892) -> (41.4344, 2.4892) centre (41.4598, 2.4892) ccw
  line L266 (41.9848, 2.4892) -> (42.3742, 1.3208)
  line L267 (40.1828, 2.4892) -> (40.8319, 1.3208)
  arc A845 (38.9636, 1.6454) -> (39.6127, 1.6454) centre (39.2881, 1.6454) ccw
  arc A846 (40.8097, 1.3085) -> (40.8541, 1.3331) centre (40.8319, 1.3208) ccw
  arc A847 (40.205, 2.5015) -> (40.1606, 2.4769) centre (40.1828, 2.4892) ccw
  arc A848 (40.8573, 2.4892) -> (40.8065, 2.4892) centre (40.8319, 2.4892) ccw
  arc A849 (44.5533, 1.8655) -> (44.5533, 1.8147) centre (44.5533, 1.8401) ccw
  arc A850 (43.233, 1.3462) -> (43.233, 1.2954) centre (43.233, 1.3208) ccw
  line L268 (44.5533, 1.8401) -> (44.2287, 1.8401)
  arc A851 (44.8551, 1.3094) -> (44.9006, 1.3322) centre (44.8779, 1.3208) ccw
  arc A852 (43.7523, 1.2954) -> (43.7523, 1.3462) centre (43.7523, 1.3208) ccw
  arc A853 (43.2076, 1.3208) -> (43.2584, 1.3208) centre (43.233, 1.3208) ccw
  arc A854 (41.4344, 1.3208) -> (41.4852, 1.3208) centre (41.4598, 1.3208) ccw
  arc A855 (38.989, 1.6454) -> (38.9382, 1.6454) centre (38.9636, 1.6454) ccw
  arc A856 (42.7878, 2.4812) -> (42.7396, 2.4972) centre (42.7637, 2.4892) ccw
  arc A857 (39.6381, 1.6454) -> (39.5873, 1.6454) centre (39.6127, 1.6454) ccw
  arc A858 (39.5873, 1.6454) -> (39.6381, 1.6454) centre (39.6127, 1.6454) ccw
  line L269 (40.1828, 1.3208) -> (40.1828, 2.4892)
  line L270 (41.33, 1.3208) -> (41.5897, 1.3208)
  line L271 (40.8319, 1.3208) -> (40.8319, 2.4892)
  arc A859 (42.0089, 2.4972) -> (41.9607, 2.4812) centre (41.9848, 2.4892) ccw
  arc A860 (43.7523, 2.4638) -> (43.7523, 2.5146) centre (43.7523, 2.4892) ccw
  arc A861 (43.233, 2.5146) -> (43.233, 2.4638) centre (43.233, 2.4892) ccw
  arc A862 (43.233, 1.9953) -> (43.233, 1.9445) centre (43.233, 1.9699) ccw
  line L272 (44.2287, 1.3208) -> (44.2287, 2.4892)
  arc A863 (44.5533, 2.4638) -> (44.5533, 2.5146) centre (44.5533, 2.4892) ccw
  arc A864 (42.3501, 1.3128) -> (42.3983, 1.3288) centre (42.3742, 1.3208) ccw
  line L273 (43.233, 1.3208) -> (43.233, 2.4892)
  arc A865 (44.2541, 2.4892) -> (44.2033, 2.4892) centre (44.2287, 2.4892) ccw
  line L274 (43.233, 1.9699) -> (43.6225, 1.9699)
  arc A866 (44.5533, 2.5146) -> (44.5533, 2.4638) centre (44.5533, 2.4892) ccw
  arc A867 (44.5533, 1.8401) -> (44.5533, 2.4892) centre (44.5533, 2.1646) ccw
  arc A868 (43.2584, 2.4892) -> (43.2076, 2.4892) centre (43.233, 2.4892) ccw
  arc A869 (38.989, 2.4892) -> (38.9382, 2.4892) centre (38.9636, 2.4892) ccw
  arc A870 (41.5897, 1.2954) -> (41.5897, 1.3462) centre (41.5897, 1.3208) ccw
  arc A871 (44.6409, 1.8514) -> (44.5955, 1.8287) centre (44.6182, 1.8401) ccw
  arc A872 (44.5533, 1.8147) -> (44.5533, 1.8655) centre (44.5533, 1.8401) ccw
  arc A873 (44.2287, 1.8655) -> (44.2287, 1.8147) centre (44.2287, 1.8401) ccw
  arc A874 (45.7157, 1.3462) -> (45.7157, 1.2954) centre (45.7157, 1.3208) ccw
  line L275 (44.2287, 2.4892) -> (44.5533, 2.4892)
  arc A875 (49.554, 1.8401) -> (49.554, 2.4892) centre (49.554, 2.1646) ccw
  arc A876 (47.6145, 1.3462) -> (47.6145, 1.2954) centre (47.6145, 1.3208) ccw
  arc A877 (50.6874, 2.4638) -> (50.6874, 2.5146) centre (50.6874, 2.4892) ccw
  arc A878 (52.1222, 2.1646) -> (52.173, 2.1646) centre (52.1476, 2.1646) ccw
  line L276 (45.8456, 1.8076) -> (45.4886, 2.0024)
  arc A879 (47.6399, 2.4892) -> (47.5891, 2.4892) centre (47.6145, 2.4892) ccw
  arc A880 (49.554, 2.5146) -> (49.554, 2.4638) centre (49.554, 2.4892) ccw
  arc A881 (45.6184, 2.5146) -> (45.6184, 2.4638) centre (45.6184, 2.4892) ccw
  arc A882 (49.204, 1.3208) -> (49.2548, 1.3208) centre (49.2294, 1.3208) ccw
  arc A883 (45.6184, 2.4892) -> (45.3587, 2.2296) centre (45.6184, 2.2295) ccw
  line L277 (49.554, 1.8401) -> (49.2294, 1.8401)
  arc A884 (49.2548, 2.4892) -> (49.204, 2.4892) centre (49.2294, 2.4892) ccw
  arc A885 (50.6874, 1.8147) -> (50.6874, 1.8655) centre (50.6874, 1.8401) ccw
  line L278 (46.7557, 2.4892) -> (47.1452, 1.3208)
  arc A886 (45.7157, 1.2954) -> (45.7157, 1.3462) centre (45.7157, 1.3208) ccw
  arc A887 (45.9105, 2.3918) -> (45.6184, 2.4892) centre (45.6184, 2.0024) ccw
  arc A888 (45.3841, 2.2296) -> (45.3333, 2.2296) centre (45.3587, 2.2296) ccw
  arc A889 (47.5891, 1.3208) -> (47.6399, 1.3208) centre (47.6145, 1.3208) ccw
  line L279 (47.6145, 1.3208) -> (48.1338, 1.3208)
  line L280 (49.2294, 2.4892) -> (49.554, 2.4892)
  arc A890 (49.554, 2.4638) -> (49.554, 2.5146) centre (49.554, 2.4892) ccw
  arc A891 (49.554, 1.8147) -> (49.554, 1.8655) centre (49.554, 1.8401) ccw
  arc A892 (45.8585, 1.8295) -> (45.8327, 1.7857) centre (45.8456, 1.8076) ccw
  arc A893 (45.3587, 2.2296) -> (45.4886, 2.0024) centre (45.6224, 2.2296) ccw
  arc A894 (45.5007, 2.0247) -> (45.4764, 1.9801) centre (45.4886, 2.0024) ccw
  arc A895 (46.0008, 1.5804) -> (45.95, 1.5804) centre (45.9754, 1.5804) ccw
  arc A896 (46.4636, 1.6383) -> (46.4636, 1.5875) centre (46.4636, 1.6129) ccw
  arc A897 (50.3374, 1.3208) -> (50.3882, 1.3208) centre (50.3628, 1.3208) ccw
  arc A898 (45.7157, 1.3208) -> (45.9754, 1.5804) centre (45.7157, 1.5805) ccw
  arc A899 (45.3333, 2.2296) -> (45.3841, 2.2296) centre (45.3587, 2.2296) ccw
  arc A900 (45.8334, 1.7853) -> (45.8577, 1.8299) centre (45.8455, 1.8076) ccw
  arc A901 (50.3628, 2.5146) -> (50.3628, 2.4638) centre (50.3628, 2.4892) ccw
  line L281 (50.6874, 1.8401) -> (50.3628, 1.8401)
  arc A902 (49.2294, 2.5146) -> (49.2294, 2.4638) centre (49.2294, 2.4892) ccw
  arc A903 (50.6874, 1.8655) -> (50.6874, 1.8147) centre (50.6874, 1.8401) ccw
  arc A904 (50.3628, 1.8655) -> (50.3628, 1.8147) centre (50.3628, 1.8401) ccw
  arc A905 (50.775, 1.8514) -> (50.7296, 1.8287) centre (50.7523, 1.8401) ccw
  arc A906 (48.1338, 1.2954) -> (48.1338, 1.3462) centre (48.1338, 1.3208) ccw
  arc A907 (45.6184, 2.4638) -> (45.6184, 2.5146) centre (45.6184, 2.4892) ccw
  arc A908 (46.3422, 1.3288) -> (46.3904, 1.3128) centre (46.3663, 1.3208) ccw
  arc A909 (45.95, 1.5804) -> (46.0008, 1.5804) centre (45.9754, 1.5804) ccw
  arc A910 (47.1211, 1.3128) -> (47.1693, 1.3288) centre (47.1452, 1.3208) ccw
  line L282 (50.3628, 1.3208) -> (50.3628, 2.4892)
  line L283 (50.3628, 2.4892) -> (50.6874, 2.4892)
  arc A911 (50.3882, 2.4892) -> (50.3374, 2.4892) centre (50.3628, 2.4892) ccw
  line L284 (51.0119, 1.3208) -> (50.7523, 1.8401)
  arc A912 (45.9754, 1.5804) -> (45.8456, 1.8076) centre (45.7117, 1.5804) ccw
  arc A913 (46.7798, 2.4972) -> (46.7316, 2.4812) centre (46.7557, 2.4892) ccw
  arc A914 (45.4757, 1.9805) -> (45.5014, 2.0242) centre (45.4885, 2.0024) ccw
  line L285 (47.0478, 1.6129) -> (46.4636, 1.6129)
  line L286 (47.6145, 2.4892) -> (47.6145, 1.3208)
  line L287 (49.2294, 1.3208) -> (49.2294, 2.4892)
  arc A915 (49.554, 1.8655) -> (49.554, 1.8147) centre (49.554, 1.8401) ccw
  line L288 (51.4985, 1.6454) -> (51.4985, 2.1646)
  arc A916 (52.1476, 2.1646) -> (51.4985, 2.1646) centre (51.8231, 2.1646) ccw
  arc A917 (50.6874, 1.8401) -> (50.6874, 2.4892) centre (50.6874, 2.1646) ccw
  line L289 (46.3663, 1.3208) -> (46.7557, 2.4892)
  arc A918 (45.8952, 2.3715) -> (45.9257, 2.4122) centre (45.9105, 2.3918) ccw
  arc A919 (46.7798, 2.4812) -> (46.7316, 2.4972) centre (46.7557, 2.4892) ccw
  arc A920 (47.0478, 1.5875) -> (47.0478, 1.6383) centre (47.0478, 1.6129) ccw
  arc A921 (50.6874, 2.5146) -> (50.6874, 2.4638) centre (50.6874, 2.4892) ccw
  arc A922 (49.2294, 1.8655) -> (49.2294, 1.8147) centre (49.2294, 1.8401) ccw
  arc A923 (50.9892, 1.3094) -> (51.0347, 1.3322) centre (51.0119, 1.3208) ccw
  arc A924 (45.3443, 1.501) -> (45.3082, 1.4652) centre (45.3262, 1.4831) ccw
  arc A925 (27.4884, 51.9684) -> (27.4884, 52.0192) centre (27.4884, 51.9938) ccw
  arc A926 (27.2542, 52.6429) -> (27.2034, 52.6429) centre (27.2288, 52.6429) ccw
  arc A927 (52.6546, 1.3462) -> (52.6546, 1.2954) centre (52.6546, 1.3208) ccw
  arc A928 (52.8888, 1.5804) -> (52.9396, 1.5804) centre (52.9142, 1.5804) ccw
  arc A929 (50.2412, 29.924) -> (50.1904, 29.924) centre (50.2158, 29.924) ccw
  line L290 (50.7351, 29.6644) -> (50.7351, 29.2749)
  line L291 (52.6546, 1.3208) -> (52.5248, 1.3208)
  arc A930 (50.2238, 31.156) -> (50.2078, 31.1078) centre (50.2158, 31.1319) ccw
  arc A931 (27.7227, 52.4482) -> (27.7735, 52.4482) centre (27.7481, 52.4482) ccw
  arc A932 (52.173, 1.6454) -> (52.1222, 1.6454) centre (52.1476, 1.6454) ccw
  line L292 (53.4819, 1.9699) -> (53.8714, 1.9699)
  arc A933 (51.5239, 2.1646) -> (51.4731, 2.1646) centre (51.4985, 2.1646) ccw
  arc A934 (52.9396, 2.4892) -> (52.8888, 2.4892) centre (52.9142, 2.4892) ccw
  line L293 (52.9142, 2.4892) -> (52.9142, 1.5804)
  arc A935 (51.5239, 1.6454) -> (51.4731, 1.6454) centre (51.4985, 1.6454) ccw
  arc A936 (54.0012, 1.2954) -> (54.0012, 1.3462) centre (54.0012, 1.3208) ccw
  arc A937 (50.7097, 29.6644) -> (50.7605, 29.6644) centre (50.7351, 29.6644) ccw
  arc A938 (27.7735, 52.6429) -> (27.7227, 52.6429) centre (27.7481, 52.6429) ccw
  arc A939 (51.4985, 1.6454) -> (52.1476, 1.6454) centre (51.8231, 1.6454) ccw
  line L294 (50.2158, 30.353) -> (51.3842, 30.7425)
  arc A940 (28.3972, 52.6175) -> (28.3972, 52.6683) centre (28.3972, 52.6429) ccw
  arc A941 (27.7481, 52.6683) -> (27.7481, 52.6175) centre (27.7481, 52.6429) ccw
  line L295 (27.7481, 52.4482) -> (27.7481, 52.6429)
  line L296 (28.3972, 52.6429) -> (28.3972, 52.2534)
  arc A942 (52.6546, 1.3208) -> (52.9142, 1.5804) centre (52.6546, 1.5804) ccw
  line L297 (54.0012, 1.3208) -> (53.4819, 1.3208)
  line L298 (51.3842, 30.7425) -> (50.2158, 31.1319)
  arc A943 (51.3762, 30.7184) -> (51.3922, 30.7666) centre (51.3842, 30.7425) ccw
  line L299 (53.4819, 1.3208) -> (53.4819, 2.4892)
  arc A944 (50.7605, 29.6644) -> (50.7097, 29.6644) centre (50.7351, 29.6644) ccw
  arc A945 (28.1376, 52.0192) -> (28.1376, 51.9684) centre (28.1376, 51.9938) ccw
  arc A946 (50.2158, 29.3003) -> (50.2158, 29.2495) centre (50.2158, 29.2749) ccw
  line L300 (50.2158, 29.2749) -> (50.2158, 29.924)
  arc A947 (28.4226, 52.2534) -> (28.3718, 52.2534) centre (28.3972, 52.2534) ccw
  line L301 (28.1376, 51.9938) -> (27.4884, 51.9938)
  arc A948 (27.4884, 52.0192) -> (27.4884, 51.9684) centre (27.4884, 51.9938) ccw
  arc A949 (50.7097, 29.2749) -> (50.7605, 29.2749) centre (50.7351, 29.2749) ccw
  arc A950 (53.4565, 1.3208) -> (53.5073, 1.3208) centre (53.4819, 1.3208) ccw
  arc A951 (28.1376, 51.9684) -> (28.1376, 52.0192) centre (28.1376, 51.9938) ccw
  arc A952 (52.1222, 1.6454) -> (52.173, 1.6454) centre (52.1476, 1.6454) ccw
  arc A953 (52.9396, 1.5804) -> (52.8888, 1.5804) centre (52.9142, 1.5804) ccw
  arc A954 (28.3718, 52.2534) -> (28.4226, 52.2534) centre (28.3972, 52.2534) ccw
  arc A955 (36.0299, 1.3462) -> (36.0299, 1.2954) centre (36.0299, 1.3208) ccw
  line L302 (53.4819, 2.4892) -> (54.0012, 2.4892)
  arc A956 (28.1376, 51.9938) -> (28.3972, 52.2534) centre (28.1376, 52.2534) ccw
  arc A957 (27.2288, 52.2534) -> (27.4884, 51.9938) centre (27.4884, 52.2534) ccw
  line L303 (52.1476, 2.1646) -> (52.1476, 1.6454)
  arc A958 (50.7351, 29.2495) -> (50.7351, 29.3003) centre (50.7351, 29.2749) ccw
  arc A959 (52.173, 2.1646) -> (52.1222, 2.1646) centre (52.1476, 2.1646) ccw
  arc A960 (54.6885, 1.3462) -> (54.6885, 1.2954) centre (54.6885, 1.3208) ccw
  arc A961 (50.1904, 29.2749) -> (50.2412, 29.2749) centre (50.2158, 29.2749) ccw
  arc A962 (50.2078, 30.3771) -> (50.2238, 30.3289) centre (50.2158, 30.353) ccw
  arc A963 (51.4731, 1.6454) -> (51.5239, 1.6454) centre (51.4985, 1.6454) ccw
  arc A964 (51.3922, 30.7184) -> (51.3762, 30.7666) centre (51.3842, 30.7425) ccw
  line L304 (50.7351, 29.2749) -> (50.2158, 29.2749)
  arc A965 (52.5248, 1.3462) -> (52.5248, 1.2954) centre (52.5248, 1.3208) ccw
  arc A966 (54.0012, 2.4638) -> (54.0012, 2.5146) centre (54.0012, 2.4892) ccw
  arc A967 (28.4226, 52.6429) -> (28.3718, 52.6429) centre (28.3972, 52.6429) ccw
  arc A968 (53.4819, 1.3462) -> (53.4819, 1.2954) centre (53.4819, 1.3208) ccw
  line L305 (27.7481, 52.6429) -> (28.3972, 52.6429)
  arc A969 (51.4731, 2.1646) -> (51.5239, 2.1646) centre (51.4985, 2.1646) ccw
  arc A970 (53.5073, 2.4892) -> (53.4565, 2.4892) centre (53.4819, 2.4892) ccw
  arc A971 (52.6546, 1.2954) -> (52.6546, 1.3462) centre (52.6546, 1.3208) ccw
  arc A972 (27.2542, 52.2534) -> (27.2034, 52.2534) centre (27.2288, 52.2534) ccw
  arc A973 (64.08, 47.4274) -> (64.1562, 47.4274) centre (64.1181, 47.4274) ccw
  arc A974 (28.1968, 7.6581) -> (28.1968, 7.7343) centre (28.1968, 7.6962) ccw
  line L306 (28.3972, 54.7567) -> (28.3972, 54.4322)
  arc A975 (28.1968, 7.6962) -> (28.5581, 8.0574) centre (28.1968, 8.0575) ccw
  arc A976 (28.0162, 7.7343) -> (28.0162, 7.6581) centre (28.0162, 7.6962) ccw
  arc A977 (27.5534, 55.1067) -> (27.5534, 55.0559) centre (27.5534, 55.0813) ccw
  line L307 (29.7163, 9.3218) -> (29.7163, 7.6962)
  arc A978 (29.6782, 7.6962) -> (29.7544, 7.6962) centre (29.7163, 7.6962) ccw
  arc A979 (29.2648, 7.7343) -> (29.2648, 7.6581) centre (29.2648, 7.6962) ccw
  arc A980 (27.2034, 54.4322) -> (27.2542, 54.4322) centre (27.2288, 54.4322) ccw
  arc A981 (29.7544, 9.3218) -> (29.6782, 9.3218) centre (29.7163, 9.3218) ccw
  arc A982 (27.5534, 55.0813) -> (27.2288, 54.7567) centre (27.5534, 54.7567) ccw
  line L308 (27.5534, 55.0813) -> (28.0726, 55.0813)
  line L309 (64.1181, 48.6918) -> (64.1181, 47.4274)
  arc A983 (65.7279, 48.2854) -> (65.3215, 48.6918) centre (65.3215, 48.2854) ccw
  arc A984 (63.7568, 47.0281) -> (63.7568, 47.1043) centre (63.7568, 47.0662) ccw
  line L310 (28.3972, 54.4322) -> (27.2288, 54.4322)
  arc A985 (63.5762, 47.1043) -> (63.5762, 47.0281) centre (63.5762, 47.0662) ccw
  line L311 (28.5581, 9.3218) -> (28.5581, 8.0574)
  line L312 (28.3972, 53.213) -> (27.2288, 53.213)
  arc A986 (65.3215, 48.7299) -> (65.3215, 48.6537) centre (65.3215, 48.6918) ccw
  arc A987 (65.3215, 48.6537) -> (65.3215, 48.7299) centre (65.3215, 48.6918) ccw
  arc A988 (64.7885, 48.3423) -> (64.861, 48.3188) centre (64.8248, 48.3306) ccw
  arc A989 (65.5661, 47.9969) -> (65.6187, 47.9417) centre (65.5924, 47.9693) ccw
  arc A990 (28.1968, 7.7343) -> (28.1968, 7.6581) centre (28.1968, 7.6962) ccw
  arc A991 (28.5962, 8.0574) -> (28.52, 8.0574) centre (28.5581, 8.0574) ccw
  arc A992 (63.7568, 47.0662) -> (64.1181, 47.4274) centre (63.7568, 47.4275) ccw
  arc A993 (65.3215, 48.6918) -> (64.8248, 48.3306) centre (65.3215, 48.1697) ccw
  arc A994 (65.5924, 47.9693) -> (65.7279, 48.2854) centre (65.2914, 48.2854) ccw
  arc A995 (28.3972, 54.4068) -> (28.3972, 54.4576) centre (28.3972, 54.4322) ccw
  arc A996 (27.2034, 54.7567) -> (27.2542, 54.7567) centre (27.2288, 54.7567) ccw
  arc A997 (28.3718, 54.4322) -> (28.4226, 54.4322) centre (28.3972, 54.4322) ccw
  arc A998 (28.4226, 54.7567) -> (28.3718, 54.7567) centre (28.3972, 54.7567) ccw
  line L313 (27.2288, 53.213) -> (28.3972, 53.8621)
  arc A999 (27.2034, 52.2534) -> (27.2542, 52.2534) centre (27.2288, 52.2534) ccw
  line L314 (28.3972, 53.8621) -> (27.2288, 53.8621)
  arc A1000 (28.3972, 54.7567) -> (28.0726, 55.0813) centre (28.0726, 54.7567) ccw
  line L315 (27.2288, 54.4322) -> (27.2288, 54.7567)
  arc A1001 (29.241, 8.9903) -> (29.2886, 8.9308) centre (29.2648, 8.9605) ccw
  arc A1002 (63.7568, 47.1043) -> (63.7568, 47.0281) centre (63.7568, 47.0662) ccw
  line L316 (29.2648, 7.6962) -> (30.1679, 7.6962)
  arc A1003 (28.4095, 53.8399) -> (28.3849, 53.8843) centre (28.3972, 53.8621) ccw
  arc A1004 (27.2542, 54.7567) -> (27.2034, 54.7567) centre (27.2288, 54.7567) ccw
  arc A1005 (27.5534, 55.0559) -> (27.5534, 55.1067) centre (27.5534, 55.0813) ccw
  line L317 (28.1968, 7.6962) -> (28.0162, 7.6962)
  arc A1006 (64.1562, 47.4274) -> (64.08, 47.4274) centre (64.1181, 47.4274) ccw
  arc A1007 (27.2288, 54.4576) -> (27.2288, 54.4068) centre (27.2288, 54.4322) ccw
  arc A1008 (28.3972, 53.1876) -> (28.3972, 53.2384) centre (28.3972, 53.213) ccw
  arc A1009 (28.0726, 55.1067) -> (28.0726, 55.0559) centre (28.0726, 55.0813) ccw
  arc A1010 (28.5962, 9.3218) -> (28.52, 9.3218) centre (28.5581, 9.3218) ccw
  arc A1011 (27.2288, 53.2384) -> (27.2288, 53.1876) centre (27.2288, 53.213) ccw
  arc A1012 (28.3972, 53.8367) -> (28.3972, 53.8875) centre (28.3972, 53.8621) ccw
  arc A1013 (28.3718, 54.7567) -> (28.4226, 54.7567) centre (28.3972, 54.7567) ccw
  arc A1014 (27.2165, 53.2352) -> (27.2411, 53.1908) centre (27.2288, 53.213) ccw
  arc A1015 (28.0726, 55.0559) -> (28.0726, 55.1067) centre (28.0726, 55.0813) ccw
  arc A1016 (28.52, 8.0574) -> (28.5962, 8.0574) centre (28.5581, 8.0574) ccw
  line L318 (27.2288, 52.2534) -> (27.2288, 52.6429)
  arc A1017 (29.7401, 9.292) -> (29.6925, 9.3516) centre (29.7163, 9.3218) ccw
  line L319 (29.2648, 8.9606) -> (29.7163, 9.3218)
  arc A1018 (30.1679, 7.6581) -> (30.1679, 7.7343) centre (30.1679, 7.6962) ccw
  arc A1019 (64.1562, 48.6918) -> (64.08, 48.6918) centre (64.1181, 48.6918) ccw
  line L320 (63.7568, 47.0662) -> (63.5762, 47.0662)
  arc A1020 (65.6898, 48.2854) -> (65.766, 48.2854) centre (65.7279, 48.2854) ccw